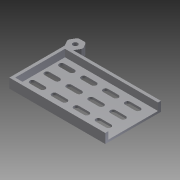
# Autodesk Inventor part: case add on sdr top
Saved by Autodesk Inventor 2012 (Build 160160000, 160)
## iProperties
Created: 2018-03-05
Part Number: case add on sdr top
Material: Default
Document SubType Name: Modeling
Designer: kanu
Density: 1 g/cm^3
Author: kanu
Autodesk Inventor part; units mm, degrees
ref_plane "YZ Plane" through (0, 0, 0) normal (1, 0, 0) x (0, 1, 0)
ref_plane "XZ Plane" through (0, 0, 0) normal (0, 1, 0) x (-1, 0, 0)
ref_plane "XY Plane" through (0, 0, 0) normal (0, 0, 1) x (1, 0, 0)
sketch "Sketch1" plane through (0, 0, 0) normal (0, 0, 1) x (1, 0, 0)
  circle A0 centre (16.5752, 43.5198) radius 1.65
  line L0 (21.3312, 42.5198) -> (19.4442, 39.2514)
  arc A1 (21.3312, 42.5198) -> (21.3312, 44.5198) centre (19.5992, 43.5198) ccw
  line L1 (19.8192, 47.1386) -> (21.3312, 44.5198)
  arc A2 (19.8192, 47.1386) -> (18.0872, 48.1386) centre (18.0872, 46.1386) ccw
  line L2 (15.0633, 48.1386) -> (18.0872, 48.1386)
  arc A3 (15.0633, 48.1386) -> (13.3312, 47.1386) centre (15.0633, 46.1386) ccw
  line L3 (11.8192, 44.5198) -> (13.3312, 47.1386)
  arc A4 (11.8192, 44.5198) -> (11.8192, 42.5198) centre (13.5513, 43.5198) ccw
  line L4 (13.7915, 39.1038) -> (11.8192, 42.5198)
  line L5 (13.7915, 39.1038) -> (13.7915, 1.2514)
  line L6 (13.7915, 1.2514) -> (79.2915, 1.2514)
  line L7 (79.2915, 1.2514) -> (79.2915, 39.2514)
  line L8 (79.2915, 39.2514) -> (19.4442, 39.2514)
  point P0 (0, 0)
  point P1 (0, 0)
  dimension "d0" = 65.5
  dimension "d1" = 38
  dimension "d3" = 37.8524
  dimension "d4" = 90
  dimension "d5" = 90
  dimension "d6" = 5.6528
  dimension "d10" = 90
  constraints: 18 end point, 8 point on circle, 5 centre point, 1 parallel, 1 point on line
  measures "d0" distance of L6.start L6.end
  measures "d1" distance of L6.end L7.end
  measures "d3" distance of L5.start L6.start
  measures "d4" angle of L6 L5
  measures "d5" angle of L7 L6
  measures "d6" horizontal distance of L5.start L0.end
  measures "d10" angle of L8 L7
extrude "Extrusion1" add sketch "Sketch1" along normal blind 1.5
sketch "Sketch2" plane through (0, 0, 0) normal (0, 0, -1) x (-1, 0, 0)
  circle A0 centre (-16.5752, 43.5198) radius 1.65 projected
  line L0 (-13.7915, 1.2514) -> (-13.7915, 39.1038) projected
  line L1 (-13.7915, 39.1038) -> (-11.8192, 42.5198) projected
  arc A1 (-11.8192, 42.5198) -> (-11.8192, 44.5198) centre (-13.5513, 43.5198) ccw projected
  line L2 (-11.8192, 44.5198) -> (-13.3312, 47.1386) projected
  arc A2 (-13.3312, 47.1386) -> (-15.0633, 48.1386) centre (-15.0633, 46.1386) ccw projected
  line L3 (-15.0633, 48.1386) -> (-18.0872, 48.1386) projected
  arc A3 (-18.0872, 48.1386) -> (-19.8192, 47.1386) centre (-18.0872, 46.1386) ccw projected
  line L4 (-19.8192, 47.1386) -> (-21.3312, 44.5198) projected
  arc A4 (-21.3312, 44.5198) -> (-21.3312, 42.5198) centre (-19.5992, 43.5198) ccw projected
  line L5 (-21.3312, 42.5198) -> (-19.4442, 39.2514) projected
  line L6 (-19.4442, 39.2514) -> (-79.2915, 39.2514) projected
  line L7 (-79.2915, 39.2514) -> (-79.2915, 1.2514) projected
  line L8 (-79.2915, 1.2514) -> (-13.7915, 1.2514) projected
  line L9 (-77.7629, 37.2514) -> (-15.7915, 37.2514)
  line L10 (-15.7915, 37.2514) -> (-15.7915, 3.2514)
  line L11 (-15.7915, 3.2514) -> (-77.7629, 3.2514)
  line L12 (-77.7629, 37.2514) -> (-79.2915, 37.2514)
  line L13 (-77.7629, 3.2514) -> (-79.2915, 3.2514)
  point P0 (0, 0)
  dimension "d11" = 2
  dimension "d12" = 2
  dimension "d13" = 2
  constraints: 10 end point, 3 perpendicular, 2 point on line, 1 horizontal, 1 parallel
  measures "d11" distance between parallel lines of L6 L9
  measures "d12" distance between parallel lines of L8 L11
  measures "d13" distance between parallel lines of L0 L10
extrude "Extrusion2" add sketch "Sketch2" against normal blind 6.5 contours L8 L7 L13 L11 L10 L9 L12 L6 L5 A4 L4 A3 L3 A2 L2 A1 L1 L0
sketch "Sketch3" plane through (0, 0, 0) normal (0, 0, -1) x (-1, 0, 0)
  line L0 (-79.2915, 39.2514) -> (-79.2915, 1.2514) projected
  line L1 (-19.4442, 39.2514) -> (-79.2915, 39.2514) projected
  line L2 (-71.2915, 33.2514) -> (-64.2915, 33.2514)
  line L3 (-64.2915, 33.2514) -> (-64.2915, 29.7514)
  line L4 (-64.2915, 29.7514) -> (-71.2915, 29.7514)
  line L5 (-71.2915, 29.7514) -> (-71.2915, 33.2514)
  circle A0 centre (-71.2915, 31.5014) radius 1.75
  circle A1 centre (-64.2915, 31.5014) radius 1.75
  point P0 (0, 0)
  dimension "d16" = 3.5
  dimension "d17" = 7
  dimension "d18" = 6
  dimension "d19" = 8
  constraints: 8 end point, 2 midpoint, 2 parallel, 1 centre point, 1 horizontal, 1 perpendicular, 1 tangent, 1 vertical alignment, 2 other
  measures "d16" distance between parallel lines of L4 L2
  measures "d17" distance of A1.centre point (-71.291, 31.501)
  measures "d18" distance between parallel lines of L1 L2
  measures "d19" distance from line of L0 point (-71.291, 31.501)
extrude "Extrusion3" cut sketch "Sketch3" against normal blind 2.5
pattern_linear "Rectangular Pattern1" count 4 spacing 15 along (-1, 0, 0) count 3 spacing 10 along (0, -1, 0) of "Extrusion3"
body "Solid1"
